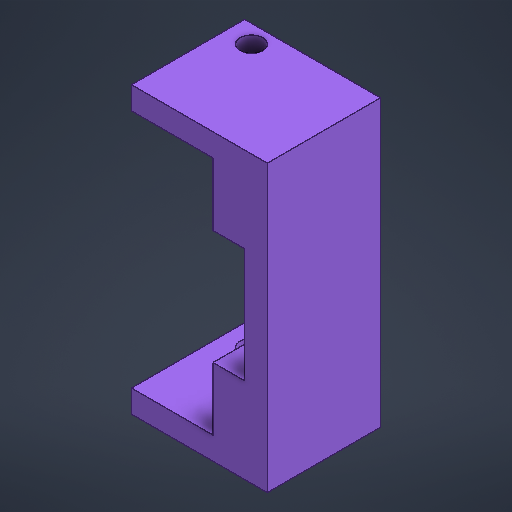
# Autodesk Inventor part: measuring_support2
Saved by Autodesk Inventor 2026.1 (Build 301233000, 233)
## iProperties
Created: 2026-01-06
Part Number: measuring_support2
Material: Generic
Document SubType Name: Modeling
Designer: emanuel
Density: 1 g/cm^3
Appearance: Violet
Author: emanuel
Autodesk Inventor part; units mm, degrees
ref_plane "YZ Plane" through (0, 0, 0) normal (1, 0, 0) x (0, 1, 0)
ref_plane "XZ Plane" through (0, 0, 0) normal (0, 1, 0) x (-1, 0, 0)
ref_plane "XY Plane" through (0, 0, 0) normal (0, 0, 1) x (1, 0, 0)
sketch "Sketch1" plane through (0, 0, 0) normal (1, 0, 0) x (0, 1, 0)
  line L0 (0, 0) -> (10.1, 0)
  line L1 (10.1, 0) -> (10.1, -10)
  line L2 (10.1, -10) -> (0, -10)
  line L3 (0, -10) -> (0, 0)
  line L4 (10.1, 0) -> (15.65, 0)
  line L5 (15.65, 0) -> (15.65, -10)
  line L6 (15.65, -10) -> (10.1, -10)
  line L7 (10.1, -10) -> (10.1, 0)
  line L8 (0, 0) -> (-5.55, 0)
  line L9 (-5.55, 0) -> (-5.55, -10)
  line L10 (-5.55, -10) -> (0, -10)
  line L11 (0, -10) -> (0, 0)
  dimension "d0" = 10.1
  dimension "d1" = 10
  dimension "d2" = 5.55
  dimension "d3" = 5.55
  constraints: 24 end point, 6 parallel, 3 horizontal, 3 perpendicular, 1 point on line
  measures "d0" distance of L1.end L2.end
  measures "d1" distance of L0.end L1.end
  measures "d2" distance of L5.end L6.end
  measures "d3" distance of L10.end L9.end
extrude "Extrusion1" add sketch "Sketch1" along normal blind 2
extrude "Extrusion2" add sketch "Sketch1" against normal blind 2.8 contours L3 L10 L9 L8 | L4 L5 L6 L1
sketch "Sketch2" plane through (2, -5.55, 0) normal (0, 0, 1) x (1, 0, 0)
  line L0 (-4.8, 21.2) -> (0, 21.2) projected
  line L1 (0, 21.2) -> (-12, 21.2)
  line L2 (-12, 21.2) -> (-12, 23.2)
  line L3 (-12, 23.2) -> (0, 23.2)
  line L4 (0, 23.2) -> (0, 21.2)
  line L5 (0, 0) -> (0, 21.2) projected
  line L6 (0, 0) -> (-12, 0)
  line L7 (-12, 0) -> (-12, -2)
  line L8 (-12, -2) -> (0, -2)
  line L9 (0, -2) -> (0, 0)
  point P0 (-2, 5.55)
  dimension "d8" = 12
  dimension "d9" = 2
  dimension "d10" = 12
  dimension "d11" = 2
  constraints: 16 end point, 4 parallel, 2 horizontal, 2 perpendicular
  measures "d8" distance of L2.end L3.end
  measures "d9" distance of L1.end L2.end
  measures "d10" distance of L8.end L7.end
  measures "d11" distance of L7.end L6.end
extrude "Extrusion3" add sketch "Sketch2" against normal blind 10
sketch "Sketch3" plane through (-10, 17.65, 0) normal (0, 1, 0) x (1, 0, 0)
  line L0 (0, 10) -> (7.2, 10) projected
  line L1 (0, 10) -> (3.2, 10)
  line L2 (3.2, 10) -> (3.2, 6.8)
  line L3 (3.2, 6.8) -> (0, 6.8)
  line L4 (0, 6.8) -> (0, 10)
  line L5 (3.2, 8.4) -> (2.2, 8.4)
  circle A0 centre (2.2, 8.4) radius 1
  point P0 (10, 0)
  dimension "d14" = 3.2
  dimension "d15" = 3.2
  dimension "d16" = 1
  constraints: 10 end point, 2 horizontal, 2 parallel, 1 coincident, 1 horizontal alignment, 1 midpoint, 1 perpendicular, 2 other
  measures "d14" distance of L2.end L3.end
  measures "d15" distance of L1.end L2.end
  measures "d16" distance of L5.start L5.end
extrude "Extrusion4" cut sketch "Sketch3" against normal up to surface (25.2 mm away) contours A0
body "Solid1"
